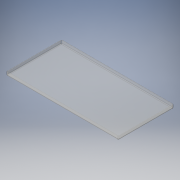
# Autodesk Inventor part: BellyPan Lexan
Saved by Autodesk Inventor 2016 (Build 200138000, 138)
## iProperties
Created: 2018-05-06
Part Number: BellyPan Lexan
Material: Polycarbonate, Clear
Document SubType Name: Sheet Metal
Designer: Kade
Density: 1.2 g/cm^3
Sheet Metal Rule: Default
Appearance: Polycarbonate - Clear
Mass: 1496.81 g
Surface Area: 7941.4 cm^2
Volume: 1247.34 cm^3
Author: Kade
Autodesk Inventor part; units mm, degrees
note: some values were not read from the file. Chosen so that the rebuilt part matches the saved one: corner form of "Plate2".
ref_plane "YZ Plane" through (0, 0, 0) normal (1, 0, 0) x (0, 1, 0)
ref_plane "XZ Plane" through (0, 0, 0) normal (0, 1, 0) x (-1, 0, 0)
ref_plane "XY Plane" through (0, 0, 0) normal (0, 0, 1) x (1, 0, 0)
sketch "Sketch1" plane through (0, 0, 0) normal (0, 1, 0) x (-1, 0, 0)
  line L0 (-50.8, 50.8) -> (768.4516, 50.8)
  line L1 (768.4516, 50.8) -> (768.4516, -352.9076)
  line L2 (768.4516, -352.9076) -> (-50.8, -352.9076)
  line L3 (-50.8, -352.9076) -> (-50.8, 50.8)
  dimension "d48" = 819.2516
  dimension "d49" = 403.7076
  measures "d48" distance of L1.end L2.end
  measures "d49" distance of L0.end L1.end
extrude "Plate1" add sketch "Sketch1" along normal blind 3.048
sketch "Sketch2" plane through (-768.4516, 0, -349.8596) normal (0, 0, -1) x (-1, 0, 0)
  line L0 (-819.2516, 0) -> (0, 0)
  line L1 (0, 0) -> (0, 25.4)
  line L2 (0, 25.4) -> (-819.2516, 25.4)
  line L3 (-819.2516, 25.4) -> (-819.2516, 0)
  constraints: 6 end point, 1 horizontal, 1 perpendicular, 1 vertical
edge flange "Flange1" height 25.4 angle 90 thickness 3.048 bend radius 3.048 thickness toward (0, 0, -1) relief tear relief width 3.048 relief depth 1.524 corner gap 3.048 corner form 2 edges at (-358.8258, 3.048, -352.9076) (-768.4516, 3.048, -151.0538) (-358.8258, 3.048, 50.8) (50.8, 3.048, -151.0538) wall of the first edge with corners at (50.8, 0, -349.8596) (-768.4516, 0, -349.8596) (-768.4516, 25.4, -349.8596) (50.8, 25.4, -349.8596)
bend "Bend1"
corner "Corner1"
equation "\"d50\" = BendReliefWidth"
equation "\"d51\" = BendReliefDepth"
equation "\"d52\" = MinimumRemnant"
equation "\"d53\" = BendRadius"
equation "\"d56\" = BendRadius"
equation "\"d57\" = CornerReliefSize"
equation "\"d58\" = GapSize"
equation "\"d59\" = JacobiRadiusSize"
equation "\"BendRadius\" = Thickness"
equation "\"BendReliefWidth\" = Thickness"
equation "\"BendReliefDepth\" = 0.5 * Thickness"
equation "\"CornerReliefSize\" = 4 * Thickness"
equation "\"MinimumRemnant\" = 2 * Thickness"
equation "\"TransitionRadius\" = BendRadius"
equation "\"JacobiRadiusSize\" = BendRadius"
equation "\"GapSize\" = Thickness"
equation "\"d47\" = BendRadius"
equation "\"Thickness\" = 3.048"
body "Solid3"
